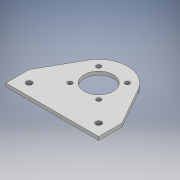
# Autodesk Inventor part: 車軸受け板
Saved by Autodesk Inventor 2017 (Build 210142000, 142)
## iProperties
Part Number: 車軸受け板
Material: 一般
Document SubType Name: Modeling
Designer: highs
Density: 1 g/cm^3
Appearance: 既定
Author: highs
Autodesk Inventor part; units mm, degrees
ref_plane "YZ Plane" through (0, 0, 0) normal (1, 0, 0) x (0, 1, 0)
ref_plane "XZ Plane" through (0, 0, 0) normal (0, 1, 0) x (-1, 0, 0)
ref_plane "XY Plane" through (0, 0, 0) normal (0, 0, 1) x (1, 0, 0)
sketch "スケッチ1" plane through (0, 0, 0) normal (0, 0, 1) x (1, 0, 0)
  line L0 (0, 0) -> (80, 0)
  line L1 (80, 0) -> (80, 20)
  line L2 (40, 0) -> (40, 90.8523) construction
  line L3 (0, 20) -> (0, 0)
  line L4 (0, 20) -> (18.2298, 52.2905)
  line L5 (61.7702, 52.2905) -> (80, 20)
  arc A0 (61.7702, 52.2905) -> (18.2298, 52.2905) centre (40, 40) ccw
  circle A1 centre (40, 40) radius 12.55
  line L6 (0, 10) -> (80, 10) construction
  circle A2 centre (10, 10) radius 2.5
  circle A3 centre (70, 10) radius 2.5
  circle A4 centre (40, 40) radius 17.5 construction
  line L7 (0, 20) -> (80, 20) construction
  line L8 (40, 40) -> (52.3744, 52.3744) construction
  circle A5 centre (52.3744, 52.3744) radius 2
  circle A6 centre (27.6256, 52.3744) radius 2
  circle A7 centre (27.6256, 27.6256) radius 2
  circle A8 centre (52.3744, 27.6256) radius 2
  dimension "d11" = 35
  dimension "d0" = 20
  dimension "d2" = 80
  dimension "d3" = 25
  dimension "d4" = 40
  dimension "d5" = 25.1
  dimension "d6" = 5
  dimension "d7" = 10
  dimension "d17" = 45
  dimension "d18" = 4
  dimension "d21" = 360
  constraints: 18 end point, 8 centre point, 3 coincident, 3 midpoint, 3 point on line, 2 horizontal, 2 point on circle, 2 tangent, 1 parallel, 1 perpendicular, 1 symmetric about line, 1 vertical, 14 other
  measures "d0" distance of L3.start L0.start
  measures "d2" distance of L0.start L0.end
  measures "d3" radius of A0
  measures "d4" distance from line of L0 A0.centre
  measures "d5" diameter of A1
  measures "d6" diameter of A2
  measures "d7" distance from line of L3 A2.centre
  measures "d17" angle of L2 L8
  measures "d18" diameter of A5
extrude "押し出し2" add sketch "スケッチ1" along normal blind 3
